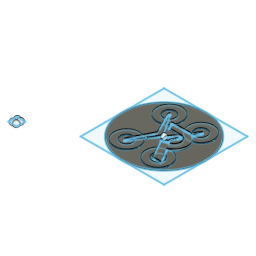
2023_02_01_DroneXR Logo Fusion360 v2 (Autodesk Fusion 360 design; units mm, degrees)
Autodesk Fusion 360 part; units mm, degrees
sketch "Esquisse1" plane through (0, 0, 0) normal (0, 0, 1) x (1, 0, 0)
  circle A0 centre (-3.2921, 4.4307) radius 1.2456
  circle A1 centre (-3.272, 4.4103) radius 2.5804
  circle A2 centre (3.328, 4.4103) radius 2.5804
  circle A3 centre (3.3079, 4.4307) radius 1.2456
  circle A4 centre (3.3079, -4.5693) radius 1.2456
  circle A5 centre (3.328, -4.5897) radius 2.5804
  circle A6 centre (-3.272, -4.5897) radius 2.5804
  circle A7 centre (-3.2921, -4.5693) radius 1.2456
  dimension "d1" = 5.1608
  dimension "d2" = 5.1608
  dimension "d3" = 5.1608
  dimension "d4" = 5.1608
  measures "d1" diameter of A1
  measures "d2" diameter of A2
  measures "d3" diameter of A6
  measures "d4" diameter of A5
sketch "Esquisse2" plane through (0, 0, 0) normal (0, 0, 1) x (1, 0, 0)
sketch "Esquisse3" plane through (0, 0, 0) normal (0, 0, 1) x (1, 0, 0)
  line L0 (-8.834, 8.7092) -> (9, 8.7092)
  line L1 (9, 8.7092) -> (9, -9)
  line L2 (9, -9) -> (-8.834, -9)
  line L3 (-8.834, -9) -> (-8.834, 8.7092)
  constraint horizontal L0
  constraint vertical L1
  constraint horizontal L2
  constraint vertical L3
extrude "Extrusion1" add sketch "Esquisse3" along normal blind 1 makes body 1
sketch "Esquisse4" plane through (0, 0, 1) normal (0, 0, 1) x (1, 0, 0)
  line L0 (163.6647, 105.2472) -> (164.171, 106.2352)
  line L1 (168.4405, 114.5503) -> (169.3629, 116.3496)
  line L2 (172.2245, 121.9555) -> (172.5459, 122.5884)
  line L3 (163.1727, 104.2862) -> (163.6647, 105.2472)
  line L4 (162.6946, 103.3518) -> (163.1727, 104.2862)
  line L5 (165.7765, 109.3648) -> (166.3413, 110.4645)
  line L6 (164.171, 106.2352) -> (164.6915, 107.2505)
  line L7 (169.3629, 116.3496) -> (169.8158, 117.2344)
  line L8 (169.8158, 117.2344) -> (170.2592, 118.1011)
  line L9 (170.2592, 118.1011) -> (170.6898, 118.944)
  line L10 (171.5009, 120.5336) -> (171.8752, 121.2685)
  line L11 (171.1047, 119.7568) -> (171.5009, 120.5336)
  line L12 (164.6915, 107.2505) -> (165.2267, 108.2936)
  line L13 (166.3413, 110.4645) -> (166.9213, 111.5932)
  line L14 (170.6898, 118.944) -> (171.1047, 119.7568)
  line L15 (165.2267, 108.2936) -> (165.7765, 109.3648)
  line L16 (167.5165, 112.7512) -> (168.4405, 114.5503)
  line L17 (171.8752, 121.2685) -> (172.2245, 121.9555)
  line L18 (166.9213, 111.5932) -> (167.5165, 112.7512)
  line L19 (169.7379, 137.8689) -> (169.0151, 139.2846)
  line L20 (158.4614, 160.0548) -> (158.1062, 160.7629)
  line L21 (156.2644, 164.4652) -> (156.0029, 164.9969)
  line L22 (158.8311, 159.3192) -> (158.4614, 160.0548)
  line L23 (175.0197, 127.5244) -> (169.7379, 137.8689)
  line L24 (156.0029, 164.9969) -> (155.7536, 165.5058)
  line L25 (153.887, 175.9712) -> (153.9857, 175.8402)
  line L26 (159.2157, 158.5552) -> (158.8311, 159.3192)
  line L27 (152.7535, 176.1782) -> (152.8565, 176.2955)
  line L28 (158.1062, 160.7629) -> (157.7652, 161.4439)
  line L29 (173.4904, 124.4603) -> (175.0197, 127.5244)
  line L30 (155.2906, 166.4578) -> (154.8728, 167.3261)
  line L31 (165.0973, 146.9651) -> (164.5114, 148.1152)
  line L32 (156.8251, 163.331) -> (156.5384, 163.9101)
  line L33 (156.5384, 163.9101) -> (156.2644, 164.4652)
  line L34 (168.3127, 140.6606) -> (167.6305, 141.9974)
  line L35 (162.8629, 151.3547) -> (162.3489, 152.3664)
  line L36 (172.5459, 122.5884) -> (172.8363, 123.1614)
  line L37 (157.7652, 161.4439) -> (157.4383, 162.0986)
  line L38 (157.4383, 162.0986) -> (157.125, 162.7274)
  line L39 (155.7536, 165.5058) -> (155.5163, 165.9926)
  line L40 (160.9087, 155.2051) -> (160.4617, 156.088)
  line L41 (161.372, 154.291) -> (160.9087, 155.2051)
  line L42 (152.4093, 174.3945) -> (152.4147, 174.7456)
  line L43 (172.8363, 123.1614) -> (173.0925, 123.6683)
  line L44 (159.6155, 157.7625) -> (159.2157, 158.5552)
  line L45 (173.0925, 123.6683) -> (173.3116, 124.1033)
  line L46 (161.852, 153.3449) -> (161.372, 154.291)
  line L47 (167.6305, 141.9974) -> (166.9681, 143.2957)
  line L48 (166.3253, 144.5559) -> (165.7018, 145.7789)
  line L49 (162.3489, 152.3664) -> (161.852, 153.3449)
  line L50 (163.9439, 149.2297) -> (163.3945, 150.3094)
  line L51 (160.4617, 156.088) -> (160.0307, 156.9403)
  line L52 (153.0203, 171.4671) -> (152.8804, 171.8403)
  line L53 (224.1626, 173.5518) -> (224.0834, 173.0993)
  line L54 (157.125, 162.7274) -> (156.8251, 163.331)
  line L55 (166.9681, 143.2957) -> (166.3253, 144.556)
  line L56 (155.5163, 165.9926) -> (155.2906, 166.4578)
  line L57 (154.8729, 167.3261) -> (154.4981, 168.1155)
  line L58 (169.0151, 139.2846) -> (168.3127, 140.6606)
  line L59 (160.0307, 156.9403) -> (159.6155, 157.7625)
  line L60 (165.7018, 145.7789) -> (165.0973, 146.9651)
  line L61 (164.5114, 148.1152) -> (163.9439, 149.2297)
  line L62 (173.3116, 124.1033) -> (173.4904, 124.4603)
  line L63 (163.3945, 150.3094) -> (162.8629, 151.3547)
  line L64 (152.4197, 174.0139) -> (152.4093, 174.3945)
  line L65 (153.8079, 176.0723) -> (153.887, 175.9712)
  line L66 (154.2397, 175.492) -> (154.3938, 175.2765)
  line L67 (223.966, 172.605) -> (223.8091, 172.0654)
  line L68 (153.6081, 170.0588) -> (153.3818, 170.5812)
  line L69 (152.671, 172.4716) -> (152.5966, 172.7394)
  line L70 (224.2047, 173.9663) -> (224.1626, 173.5518)
  line L71 (154.1035, 175.6802) -> (154.2397, 175.492)
  line L72 (152.4147, 174.7456) -> (152.4355, 175.0662)
  line L73 (223.6117, 171.4766) -> (223.3725, 170.835)
  line L74 (159.2102, 168.2167) -> (159.9788, 167.0685)
  line L75 (223.3725, 170.835) -> (223.0905, 170.1367)
  line L76 (152.4464, 173.6048) -> (152.4197, 174.0139)
  line L77 (223.0905, 170.1367) -> (222.7643, 169.378)
  line L78 (154.4981, 168.1155) -> (154.164, 168.8308)
  line L79 (152.5214, 175.6122) -> (152.5854, 175.8355)
  line L80 (152.5854, 175.8355) -> (152.663, 176.0245)
  line L81 (153.0982, 176.4172) -> (153.2358, 176.4197)
  line L82 (152.9716, 176.3755) -> (153.0982, 176.4172)
  line L83 (152.4967, 173.2035) -> (152.4464, 173.6048)
  line L84 (155.178, 174.1567) -> (155.4132, 173.8165)
  line L85 (154.3938, 175.2765) -> (154.5652, 175.0343)
  line L86 (154.9579, 174.4736) -> (155.178, 174.1567)
  line L87 (222.7643, 169.378) -> (222.3929, 168.5553)
  line L88 (155.9267, 173.0696) -> (156.4938, 172.2394)
  line L89 (152.7648, 172.1735) -> (152.671, 172.4716)
  line L90 (153.9857, 175.8402) -> (154.1035, 175.6802)
  line L91 (160.7744, 165.8763) -> (161.5923, 164.6467)
  line L92 (153.3841, 176.3819) -> (153.5425, 176.3029)
  line L93 (156.4938, 172.2394) -> (157.1102, 171.3324)
  line L94 (157.7714, 170.3553) -> (158.4729, 169.3145)
  line L95 (152.4355, 175.0662) -> (152.4712, 175.3554)
  line L96 (155.4132, 173.8165) -> (155.9267, 173.0696)
  line L97 (159.9788, 167.0685) -> (160.7744, 165.8763)
  line L98 (157.1102, 171.3324) -> (157.7714, 170.3553)
  line L99 (153.2358, 176.4197) -> (153.3841, 176.3819)
  line L100 (153.7488, 176.1428) -> (153.8079, 176.0723)
  line L101 (154.5652, 175.0343) -> (154.7535, 174.7664)
  line L102 (152.663, 176.0245) -> (152.7535, 176.1782)
  line L103 (153.3818, 170.5812) -> (153.1866, 171.049)
  line L104 (218.717, 161.3608) -> (218.4584, 161.0444)
  line L105 (154.7535, 174.7664) -> (154.9579, 174.4736)
  line L106 (152.4712, 175.3554) -> (152.5214, 175.6122)
  line L107 (153.7105, 176.1818) -> (153.7488, 176.1428)
  line L108 (224.1826, 174.6965) -> (224.211, 174.3467)
  line L109 (153.1866, 171.049) -> (153.0203, 171.4671)
  line L110 (217.6792, 160.635) -> (217.3833, 160.654)
  line L111 (153.5425, 176.3029) -> (153.7105, 176.1818)
  line L112 (158.4729, 169.3145) -> (159.2102, 168.2167)
  line L113 (161.5923, 164.6467) -> (162.4282, 163.3863)
  line L114 (152.5966, 172.7394) -> (152.4967, 173.2035)
  line L115 (153.8681, 169.477) -> (153.6081, 170.0588)
  line L116 (224.0262, 175.3196) -> (224.1206, 175.0196)
  line L117 (219.6742, 171.3631) -> (220.1184, 172.0026)
  line L118 (224.211, 174.3467) -> (224.2047, 173.9663)
  line L119 (224.0834, 173.0993) -> (223.966, 172.605)
  line L120 (152.8565, 176.2955) -> (152.9716, 176.3755)
  line L121 (215.1574, 161.5826) -> (213.5466, 162.3277)
  line L122 (220.5449, 172.6114) -> (220.951, 173.1861)
  line L123 (224.1206, 175.0196) -> (224.1826, 174.6965)
  line L124 (221.975, 167.6647) -> (221.5095, 166.7027)
  line L125 (223.8091, 172.0654) -> (223.6117, 171.4766)
  line L126 (223.8592, 175.6869) -> (224.0262, 175.3196)
  line L127 (220.7264, 165.1271) -> (220.4764, 164.6246)
  line L128 (223.0053, 175.951) -> (223.155, 176.1234)
  line L129 (152.8804, 171.8403) -> (152.7648, 172.1735)
  line L130 (154.164, 168.8308) -> (153.8681, 169.477)
  line L131 (220.2437, 164.1569) -> (220.0272, 163.723)
  line L132 (218.2062, 160.8228) -> (217.95, 160.6888)
  line L133 (221.3341, 173.723) -> (221.6917, 174.2185)
  line L134 (223.261, 176.2295) -> (223.3207, 176.2656)
  line L135 (219.6372, 162.9533) -> (219.4611, 162.6155)
  line L136 (218.2607, 169.2967) -> (218.7427, 170.0066)
  line L137 (217.95, 160.6888) -> (217.6792, 160.635)
  line L138 (222.585, 175.4213) -> (222.8144, 175.7157)
  line L139 (223.3975, 176.2463) -> (223.4833, 176.191)
  line L140 (216.2392, 161.0739) -> (215.7372, 161.3103)
  line L141 (219.1402, 162.0295) -> (218.9927, 161.7795)
  line L142 (219.2147, 170.6966) -> (219.6742, 171.3631)
  line L143 (221.6917, 174.2185) -> (222.0211, 174.6691)
  line L144 (223.6706, 175.9877) -> (223.8592, 175.6869)
  line L145 (221.5095, 166.7027) -> (220.9953, 165.6653)
  line L146 (218.7427, 170.0066) -> (219.2147, 170.6966)
  line L147 (222.8144, 175.7157) -> (223.0053, 175.951)
  line L148 (223.4833, 176.191) -> (223.5753, 176.1035)
  line L149 (220.951, 173.1861) -> (221.3341, 173.723)
  line L150 (220.4764, 164.6246) -> (220.2437, 164.1569)
  line L151 (218.9927, 161.7795) -> (218.852, 161.5569)
  line L152 (217.3833, 160.654) -> (217.0516, 160.7384)
  line L153 (220.0272, 163.723) -> (219.8255, 163.3221)
  line L154 (220.9953, 165.6653) -> (220.7264, 165.1271)
  line L155 (219.4611, 162.6155) -> (219.2959, 162.3079)
  line L156 (215.7372, 161.3103) -> (215.1574, 161.5826)
  line L157 (223.3207, 176.2656) -> (223.3975, 176.2463)
  line L158 (222.0211, 174.6691) -> (222.3197, 175.0712)
  line L159 (222.3929, 168.5553) -> (221.975, 167.6647)
  line L160 (217.0516, 160.7384) -> (216.6738, 160.8808)
  line L161 (222.3197, 175.0712) -> (222.5851, 175.4213)
  line L162 (218.4584, 161.0444) -> (218.2062, 160.8228)
  line L163 (213.5466, 162.3277) -> (218.2607, 169.2967)
  line L164 (216.6738, 160.8808) -> (216.2392, 161.0739)
  line L165 (220.1184, 172.0026) -> (220.5449, 172.6114)
  line L166 (223.155, 176.1234) -> (223.261, 176.2295)
  line L167 (223.5753, 176.1035) -> (223.6706, 175.9877)
  line L168 (219.8255, 163.3221) -> (219.6372, 162.9532)
  line L169 (218.852, 161.5569) -> (218.717, 161.3608)
  line L170 (219.2959, 162.3079) -> (219.1402, 162.0295)
  line L171 (226.9033, 88.3318) -> (227.2681, 87.7236)
  line L172 (222.1093, 156.076) -> (222.1115, 156.0742)
  line L173 (229.0186, 84.7682) -> (229.1794, 84.4974)
  line L174 (229.7465, 83.5555) -> (230.1781, 82.847)
  line L175 (231.1091, 81.3361) -> (232.0404, 79.8471)
  line L176 (216.8371, 104.8931) -> (216.9864, 104.6566)
  line L177 (219.9288, 99.8599) -> (220.3805, 99.1177)
  line L178 (227.9081, 86.6529) -> (228.1775, 86.2)
  line L179 (216.4685, 105.4941) -> (216.8371, 104.8931)
  line L180 (215.9806, 106.7639) -> (215.9168, 106.6982)
  line L181 (217.4117, 103.9725) -> (217.682, 103.5343)
  line L182 (215.8945, 106.6574) -> (215.9122, 106.5723)
  line L183 (226.5126, 88.9823) -> (226.9033, 88.3318)
  line L184 (228.1775, 86.2) -> (228.4095, 85.8085)
  line L185 (220.3805, 99.1177) -> (220.8467, 98.3511)
  line L186 (222.7974, 95.136) -> (223.784, 93.5059)
  line L187 (227.6039, 87.1624) -> (227.9081, 86.6529)
  line L188 (216.0528, 106.2499) -> (216.1679, 106.027)
  line L189 (221.8105, 96.7638) -> (222.7974, 95.136)
  line L190 (215.9168, 106.6982) -> (215.8945, 106.6574)
  line L191 (228.601, 85.4829) -> (228.7493, 85.2282)
  line L192 (219.4943, 100.573) -> (219.9288, 99.8599)
  line L193 (218.6887, 101.8926) -> (219.08, 101.2521)
  line L194 (229.3555, 84.2032) -> (229.7465, 83.5555)
  line L195 (226.0988, 89.6702) -> (226.5126, 88.9823)
  line L196 (229.1794, 84.4974) -> (229.3555, 84.2032)
  line L197 (202.7538, 99.6614) -> (201.9677, 101.0015)
  line L198 (227.2681, 87.7236) -> (227.6039, 87.1624)
  arc A0 (214.7629, 79.2757) -> (208.7557, 89.4625) centre (-17229.0104, -10200.5977) ccw
  line L199 (196.5103, 110.3428) -> (195.947, 111.3124)
  line L200 (194.8163, 119.1078) -> (195.4814, 119.1331)
  line L201 (230.1781, 82.847) -> (231.1091, 81.3361)
  line L202 (224.7475, 91.9115) -> (225.2134, 91.1396)
  line L203 (205.2271, 95.4521) -> (204.3845, 96.885)
  line L204 (218.5038, 76.1852) -> (216.7108, 75.9697)
  line L205 (217.1789, 104.3482) -> (217.4117, 103.9725)
  line L206 (191.688, 118.7768) -> (191.6308, 118.8958)
  line L207 (215.9663, 106.4341) -> (216.0528, 106.2499)
  line L208 (193.6407, 119.06) -> (194.2012, 119.0833)
  line L209 (206.9617, 92.5056) -> (206.0865, 93.9918)
  line L210 (201.9677, 101.0015) -> (201.2023, 102.3072)
  line L211 (199.4034, 119.2664) -> (200.276, 119.2932)
  line L212 (228.8746, 85.0127) -> (229.0186, 84.7682)
  line L213 (218.3234, 102.4896) -> (218.6887, 101.8926)
  line L214 (220.8467, 98.3511) -> (221.8105, 96.7638)
  line L215 (200.276, 119.2932) -> (208.8366, 119.5514)
  line L216 (215.9122, 106.5723) -> (215.9663, 106.4341)
  line L217 (192.891, 116.6136) -> (192.5931, 117.1381)
  line L218 (191.7878, 118.5859) -> (191.688, 118.7768)
  line L219 (225.2134, 91.1396) -> (225.6647, 90.3909)
  line L220 (216.1679, 106.027) -> (216.4685, 105.4941)
  line L221 (224.4113, 76.3855) -> (223.064, 76.3651)
  line L222 (193.2256, 116.0275) -> (192.891, 116.6136)
  line L223 (193.5958, 115.3815) -> (193.2256, 116.0275)
  line L224 (192.3329, 117.5993) -> (192.1112, 117.9955)
  line L225 (196.9443, 119.1856) -> (197.7332, 119.2124)
  line L226 (216.7108, 75.9697) -> (214.7629, 79.2757)
  line L227 (207.8518, 90.9952) -> (206.9617, 92.5056)
  line L228 (197.1024, 109.3251) -> (196.5103, 110.3428)
  line L229 (200.4588, 103.5769) -> (199.738, 104.8089)
  line L230 (232.0404, 79.8471) -> (234.2115, 76.4068)
  line L231 (192.5931, 117.1381) -> (192.3329, 117.5993)
  line L232 (217.9868, 103.0385) -> (218.3234, 102.4896)
  line L233 (228.7493, 85.2282) -> (228.8746, 85.0127)
  line L234 (234.2115, 76.4068) -> (227.2542, 76.4037)
  line L235 (217.682, 103.5343) -> (217.9868, 103.0385)
  line L236 (228.4095, 85.8085) -> (228.601, 85.4829)
  line L237 (223.784, 93.5059) -> (224.7475, 91.9115)
  line L238 (222.5957, 111.1484) -> (222.5957, 111.1484)
  line L239 (219.08, 101.2521) -> (219.4943, 100.573)
  line L240 (194.0006, 114.6773) -> (193.5958, 115.3815)
  line L241 (216.9864, 104.6566) -> (217.1789, 104.3482)
  line L242 (225.6647, 90.3909) -> (226.0988, 89.6702)
  line L243 (198.3687, 107.1527) -> (197.7222, 108.2612)
  line L244 (192.0329, 118.9807) -> (192.3308, 118.9981)
  line L245 (194.0711, 161.5559) -> (195.3383, 161.5737)
  line L246 (199.738, 104.8089) -> (199.041, 106.0014)
  line L247 (177.1219, 161.4007) -> (178.1749, 161.4193)
  line L248 (196.1923, 119.1591) -> (196.9443, 119.1856)
  line L249 (206.0865, 93.9918) -> (205.2271, 95.4521)
  line L250 (199.041, 106.0014) -> (198.3687, 107.1527)
  line L251 (219.749, 76.2691) -> (219.3497, 76.2492)
  line L252 (194.2012, 119.0833) -> (194.8163, 119.1078)
  line L253 (178.3207, 149.9378) -> (178.1604, 150.2288)
  line L254 (219.006, 76.2285) -> (218.7226, 76.2071)
  line L255 (193.1392, 119.0379) -> (193.6407, 119.06)
  line L256 (220.1996, 76.288) -> (219.749, 76.2691)
  line L257 (172.5687, 161.2483) -> (172.7534, 161.2614)
  line L258 (191.6308, 118.8958) -> (191.6172, 118.9413)
  line L259 (194.4392, 113.9166) -> (194.0006, 114.6773)
  line L260 (191.8117, 118.9654) -> (192.0329, 118.9807)
  line L261 (195.947, 111.3124) -> (195.4134, 112.2324)
  line L262 (191.6172, 118.9413) -> (191.6716, 118.9522)
  line L263 (204.3845, 96.885) -> (203.5598, 98.2887)
  line L264 (223.064, 76.3651) -> (221.8139, 76.3382)
  line L265 (191.9292, 118.3249) -> (191.7878, 118.5859)
  line L266 (192.3308, 118.9981) -> (192.7011, 119.0172)
  line L267 (225.82, 76.3987) -> (224.4113, 76.3855)
  line L268 (192.7011, 119.0172) -> (193.1392, 119.0379)
  line L269 (218.7226, 76.2071) -> (218.5038, 76.1852)
  line L270 (221.8139, 76.3382) -> (221.2365, 76.3227)
  line L271 (191.6716, 118.9522) -> (191.8117, 118.9654)
  line L272 (197.7222, 108.2612) -> (197.1024, 109.3251)
  line L273 (195.4814, 119.1331) -> (196.1923, 119.1591)
  line L274 (192.1112, 117.9955) -> (191.9292, 118.3249)
  line L275 (220.6969, 76.3059) -> (220.1996, 76.288)
  line L276 (219.3497, 76.2492) -> (219.006, 76.2285)
  line L277 (194.9104, 113.101) -> (194.4392, 113.9166)
  line L278 (197.7332, 119.2124) -> (198.5543, 119.2394)
  line L279 (227.2542, 76.4037) -> (225.82, 76.3987)
  line L280 (195.4134, 112.2324) -> (194.9104, 113.101)
  line L281 (198.5543, 119.2394) -> (199.4034, 119.2664)
  line L282 (221.2365, 76.3227) -> (220.6969, 76.3059)
  line L283 (208.7557, 89.4625) -> (207.8518, 90.9952)
  line L284 (201.2023, 102.3072) -> (200.4588, 103.5769)
  line L285 (203.5598, 98.2887) -> (202.7538, 99.6614)
  line L286 (193.797, 147.6841) -> (179.5416, 147.6841)
  line L287 (185.805, 161.4888) -> (188.6273, 161.5026)
  line L288 (180.4964, 161.4512) -> (181.7509, 161.464)
  line L289 (173.7915, 161.3121) -> (174.1215, 161.3242)
  line L290 (192.7575, 161.5397) -> (194.0711, 161.5559)
  line L291 (173.1381, 159.2178) -> (172.9437, 159.5778)
  line L292 (172.9437, 159.5778) -> (172.7668, 159.9083)
  line L293 (172.969, 161.2743) -> (173.2144, 161.2871)
  line L294 (172.7668, 159.9083) -> (172.6089, 160.2069)
  line L295 (173.574, 158.4203) -> (173.3486, 158.8311)
  line L296 (177.33, 151.7233) -> (177.0846, 152.1627)
  line L297 (191.4064, 161.5254) -> (192.7575, 161.5397)
  line L298 (172.1948, 161.0294) -> (172.1526, 161.129)
  line L299 (172.4157, 161.235) -> (172.5687, 161.2483)
  line L300 (172.2082, 161.2081) -> (172.2952, 161.2216)
  line L301 (174.8725, 156.095) -> (174.3243, 157.0689)
  line L302 (173.2144, 161.2871) -> (173.4889, 161.2997)
  line L303 (176.1501, 161.3806) -> (177.1219, 161.4007)
  line L304 (176.5616, 153.0966) -> (176.0085, 154.0813)
  line L305 (183.0585, 161.4747) -> (184.4122, 161.483)
  line L306 (173.8126, 157.9879) -> (173.574, 158.4203)
  line L307 (172.6089, 160.2069) -> (172.4713, 160.4709)
  line L308 (175.2664, 161.3589) -> (176.1501, 161.3806)
  line L309 (172.1526, 161.129) -> (172.1379, 161.1809)
  line L310 (179.5416, 147.6841) -> (178.5713, 149.4789)
  line L311 (178.4583, 149.6867) -> (178.3207, 149.9378)
  line L312 (177.0846, 152.1627) -> (176.5616, 153.0966)
  line L313 (174.1215, 161.3242) -> (174.4779, 161.3361)
  line L314 (177.9793, 150.5562) -> (177.7792, 150.9167)
  line L315 (173.3487, 158.8311) -> (173.1381, 159.2178)
  line L316 (173.4889, 161.2997) -> (173.7915, 161.3121)
  line L317 (178.1749, 161.4193) -> (179.3021, 161.4362)
  line L318 (177.7792, 150.9167) -> (177.5622, 151.3069)
  line L319 (174.3243, 157.0689) -> (173.8126, 157.9879)
  line L320 (195.3383, 161.5737) -> (196.5501, 161.5929)
  line L321 (172.4713, 160.4709) -> (172.3555, 160.6978)
  line L322 (184.4122, 161.483) -> (185.805, 161.4888)
  line L323 (178.5713, 149.4789) -> (178.4583, 149.6867)
  line L324 (178.1604, 150.2288) -> (177.9793, 150.5562)
  line L325 (175.4404, 155.0898) -> (174.8725, 156.095)
  line L326 (172.3555, 160.6978) -> (172.2629, 160.8848)
  line L327 (181.7509, 161.464) -> (183.0585, 161.4747)
  line L328 (172.2629, 160.8848) -> (172.1948, 161.0294)
  line L329 (172.1379, 161.1809) -> (172.1554, 161.1946)
  line L330 (208.0524, 147.6841) -> (193.797, 147.6841)
  line L331 (172.1554, 161.1946) -> (172.2082, 161.2081)
  line L332 (176.0085, 154.0813) -> (175.4404, 155.0898)
  line L333 (172.7534, 161.2614) -> (172.969, 161.2743)
  line L334 (172.2952, 161.2216) -> (172.4157, 161.235)
  line L335 (177.5622, 151.3069) -> (177.33, 151.7233)
  line L336 (179.3021, 161.4362) -> (180.4964, 161.4511)
  line L337 (203.5703, 122.4171) -> (203.3147, 122.3953)
  line L338 (200.0392, 122.2837) -> (198.9757, 122.2783)
  line L339 (191.9008, 126.4962) -> (191.8147, 127.2457)
  line L340 (201.0796, 161.694) -> (201.4673, 161.7063)
  line L341 (208.3592, 162.0749) -> (208.7907, 162.0839)
  line L342 (202.3163, 122.339) -> (201.9151, 122.3237)
  line L343 (206.6371, 161.9991) -> (207.2866, 162.0325)
  line L344 (201.4673, 161.7063) -> (201.8277, 161.7187)
  line L345 (210.074, 162.01) -> (210.1859, 161.9717)
  line L346 (207.8592, 162.0577) -> (208.3592, 162.0749)
  line L347 (204.1359, 122.516) -> (204.0683, 122.4898)
  line L348 (208.2588, 140.4356) -> (208.0552, 140.0209)
  line L349 (208.4402, 140.8074) -> (208.2588, 140.4356)
  line L350 (207.3325, 138.5613) -> (207.0612, 138.0169)
  line L351 (198.9757, 122.2783) -> (193.668, 122.2783)
  line L352 (209.9196, 162.0405) -> (210.074, 162.01)
  line L353 (201.8277, 161.7187) -> (202.1599, 161.7313)
  line L354 (192.7247, 124.1308) -> (192.3558, 124.9384)
  line L355 (203.3147, 122.3953) -> (203.0188, 122.3749)
  line L356 (202.9755, 161.7696) -> (203.1833, 161.7825)
  line L357 (202.7349, 161.7568) -> (202.9755, 161.7696)
  line L358 (203.1833, 161.7825) -> (204.1837, 161.8492)
  line L359 (197.6977, 161.6135) -> (198.7721, 161.6353)
  line L360 (174.4779, 161.3361) -> (175.2664, 161.3589)
  line L361 (205.0899, 161.9075) -> (205.9063, 161.9574)
  line L362 (203.0188, 122.3749) -> (202.685, 122.3561)
  line L363 (207.2866, 162.0325) -> (207.8592, 162.0577)
  line L364 (209.8624, 143.7944) -> (208.7282, 141.4055)
  line L365 (201.6983, 127.4328) -> (202.8572, 125.1202)
  line L366 (200.6658, 161.6818) -> (201.0796, 161.694)
  line L367 (209.1583, 162.0849) -> (209.4661, 162.078)
  line L368 (208.7907, 162.0839) -> (209.1583, 162.0849)
  line L369 (204.6462, 133.2246) -> (201.6983, 127.4328)
  line L370 (208.5973, 141.1321) -> (208.4402, 140.8074)
  line L371 (204.1837, 161.8492) -> (205.0899, 161.9075)
  line L372 (207.8315, 139.5675) -> (207.5899, 139.0796)
  line L373 (201.4841, 122.3104) -> (201.0261, 122.2992)
  line L374 (201.0261, 122.2992) -> (200.0392, 122.2837)
  line L375 (193.668, 122.2783) -> (192.7247, 124.1308)
  line L376 (205.9063, 161.9574) -> (206.6371, 161.9991)
  line L377 (204.0683, 122.4898) -> (203.9498, 122.4645)
  arc A1 (202.8572, 125.1202) -> (204.1498, 122.543) centre (974.9031, 510.7212) ccw
  line L378 (202.1599, 161.7313) -> (202.4627, 161.744)
  line L379 (202.6851, 122.3561) -> (202.3163, 122.339)
  line L380 (188.6273, 161.5026) -> (191.4064, 161.5254)
  line L381 (209.7184, 162.0632) -> (209.9197, 162.0405)
  line L382 (202.4627, 161.744) -> (202.7349, 161.7568)
  line L383 (196.5501, 161.5929) -> (197.6977, 161.6135)
  line L384 (207.5899, 139.0796) -> (207.3325, 138.5613)
  line L385 (209.4661, 162.078) -> (209.7184, 162.0632)
  line L386 (205.8802, 135.662) -> (204.6462, 133.2246)
  line L387 (208.7282, 141.4055) -> (208.5973, 141.1321)
  line L388 (204.1498, 122.543) -> (204.1359, 122.516)
  line L389 (203.9498, 122.4645) -> (203.7829, 122.4402)
  line L390 (198.7721, 161.6353) -> (199.7644, 161.6581)
  line L391 (203.7829, 122.4402) -> (203.5703, 122.4171)
  line L392 (208.0552, 140.0209) -> (207.8316, 139.5675)
  line L393 (207.0612, 138.0169) -> (205.8802, 135.662)
  line L394 (201.9151, 122.3237) -> (201.4841, 122.3104)
  line L395 (192.3558, 124.9384) -> (192.0812, 125.727)
  line L396 (195.0358, 134.222) -> (195.4588, 134.8733)
  line L397 (205.8598, 145.5476) -> (206.1334, 145.5309)
  line L398 (193.9038, 132.4625) -> (194.2556, 133.0124)
  line L399 (193.0347, 131.0846) -> (193.2906, 131.4943)
  line L400 (192.4137, 130.0412) -> (192.5031, 130.2041)
  line L401 (195.8999, 135.5497) -> (196.8257, 136.961)
  line L402 (192.8163, 130.7301) -> (193.0347, 131.0846)
  line L403 (197.7911, 138.4216) -> (202.5328, 145.567)
  line L404 (192.0812, 125.727) -> (191.9008, 126.4962)
  line L405 (204.8933, 145.567) -> (205.2422, 145.565)
  line L406 (207.0511, 145.3969) -> (207.4389, 145.2811)
  line L407 (194.6339, 133.6003) -> (195.0358, 134.222)
  line L408 (206.6225, 145.4785) -> (207.0511, 145.3969)
  line L409 (183.6889, 131.0836) -> (183.8612, 130.806)
  line L410 (192.6382, 130.4351) -> (192.8163, 130.7301)
  line L411 (192.5031, 130.2041) -> (192.6382, 130.4351)
  line L412 (199.7644, 161.6581) -> (200.6658, 161.6819)
  line L413 (202.5328, 145.567) -> (204.8933, 145.567)
  line L414 (206.1334, 145.5309) -> (206.6225, 145.4785)
  line L415 (170.0216, 151.9137) -> (170.6134, 151.0188)
  line L416 (208.558, 144.6807) -> (209.8624, 143.7944)
  line L417 (184.2074, 130.2251) -> (184.2709, 130.1079)
  line L418 (192.1224, 129.3733) -> (192.4137, 130.0412)
  line L419 (184.2709, 130.1079) -> (184.4283, 129.7709)
  line L420 (167.4946, 155.7333) -> (168.1507, 154.7418)
  line L421 (205.5636, 145.5588) -> (205.8598, 145.5476)
  line L422 (171.7504, 149.2991) -> (172.2959, 148.4737)
  line L423 (191.823, 127.9753) -> (191.9255, 128.6846)
  line L424 (193.2906, 131.4943) -> (193.5812, 131.9551)
  line L425 (205.2422, 145.565) -> (205.5636, 145.5587)
  line L426 (183.8612, 130.806) -> (184.0041, 130.5718)
  line L427 (178.0872, 139.6955) -> (178.7787, 138.6438)
  line L428 (194.2556, 133.0124) -> (194.6339, 133.6003)
  line L429 (193.5812, 131.9551) -> (193.9038, 132.4625)
  line L430 (207.4389, 145.2811) -> (207.806, 145.1264)
  line L431 (207.8061, 145.1264) -> (208.1725, 144.9278)
  line L432 (208.1724, 144.9278) -> (208.5581, 144.6807)
  line L433 (195.4588, 134.8733) -> (195.8999, 135.5497)
  line L434 (191.9255, 128.6846) -> (192.1224, 129.3733)
  line L435 (184.119, 130.3789) -> (184.2074, 130.2251)
  line L436 (191.8147, 127.2457) -> (191.823, 127.9753)
  line L437 (196.8257, 136.961) -> (197.7911, 138.4216)
  line L438 (182.8144, 122.2968) -> (182.5222, 121.842)
  line L439 (182.6753, 132.6755) -> (182.9803, 132.2008)
  line L440 (156.4772, 82.9931) -> (156.0798, 82.4174)
  line L441 (183.6666, 123.652) -> (183.5034, 123.3863)
  line L442 (184.8223, 127.0956) -> (184.711, 126.2769)
  line L443 (183.7946, 123.8662) -> (183.6666, 123.652)
  line L444 (158.3035, 85.6556) -> (157.8137, 84.9395)
  line L445 (153.8154, 79.2221) -> (153.7313, 79.1199)
  line L446 (153.5283, 78.9933) -> (153.3816, 78.9418)
  line L447 (184.0041, 130.5718) -> (184.119, 130.3789)
  line L448 (174.3295, 145.3952) -> (174.8017, 144.6799)
  line L449 (183.25, 131.7788) -> (183.4857, 131.4072)
  line L450 (176.5513, 142.0275) -> (177.3452, 140.8226)
  line L451 (166.822, 156.7497) -> (167.4946, 155.7333)
  line L452 (183.4857, 131.4072) -> (183.6889, 131.0836)
  line L453 (181.0705, 135.1469) -> (181.5324, 134.4386)
  line L454 (172.8264, 147.6709) -> (173.3421, 146.8904)
  line L455 (181.9528, 133.7922) -> (182.3332, 133.2052)
  line L456 (180.5657, 135.9193) -> (181.0705, 135.1469)
  line L457 (171.1896, 150.1474) -> (171.7504, 149.2991)
  line L458 (166.1326, 157.7912) -> (166.822, 156.7497)
  line L459 (153.7313, 79.1199) -> (153.6849, 79.0747)
  line L460 (177.3452, 140.8226) -> (178.0872, 139.6955)
  line L461 (184.8349, 127.9007) -> (184.841, 127.5006)
  line L462 (153.3816, 78.9418) -> (153.2449, 78.9202)
  line L463 (178.1814, 115.2262) -> (177.6314, 114.3964)
  line L464 (174.8017, 144.6799) -> (175.704, 143.3125)
  line L465 (156.0798, 82.4174) -> (155.7084, 81.8811)
  line L466 (175.704, 143.3125) -> (176.5513, 142.0275)
  line L467 (180.0165, 136.758) -> (180.5657, 135.9193)
  line L468 (184.1962, 124.6495) -> (183.7946, 123.8662)
  line L469 (170.6134, 151.0188) -> (171.1896, 150.1474)
  line L470 (172.2959, 148.4737) -> (172.8264, 147.6709)
  line L471 (182.9803, 132.2008) -> (183.25, 131.7788)
  line L472 (163.2041, 162.2147) -> (163.9622, 161.0697)
  line L473 (168.1507, 154.7418) -> (168.7904, 153.7749)
  line L474 (164.7029, 159.9509) -> (165.4263, 158.8582)
  line L475 (184.5602, 129.4195) -> (184.6667, 129.0552)
  line L476 (173.843, 146.132) -> (174.3295, 145.3952)
  line L477 (178.7787, 138.6438) -> (179.4213, 137.6655)
  line L478 (173.3421, 146.8904) -> (173.843, 146.132)
  line L479 (165.4263, 158.8582) -> (166.1326, 157.7912)
  line L480 (182.3332, 133.2052) -> (182.6753, 132.6756)
  line L481 (169.414, 152.8323) -> (170.0216, 151.9137)
  line L482 (184.841, 127.5006) -> (184.8223, 127.0956)
  line L483 (181.5324, 134.4386) -> (181.9528, 133.7922)
  line L484 (180.1942, 118.2748) -> (179.7215, 117.5568)
  line L485 (182.5222, 121.842) -> (182.2006, 121.3444)
  line L486 (159.3421, 87.1781) -> (158.8133, 86.4023)
  line L487 (163.9622, 161.0697) -> (164.7029, 159.9509)
  line L488 (179.4213, 137.6655) -> (180.0165, 136.7581)
  line L489 (162.4282, 163.3863) -> (163.2041, 162.2147)
  line L490 (168.7904, 153.7749) -> (169.414, 152.8323)
  line L491 (184.7479, 128.6796) -> (184.8039, 128.2942)
  line L492 (157.072, 92.255) -> (157.6655, 93.4421)
  line L493 (161.6234, 90.5355) -> (160.4519, 88.8094)
  line L494 (168.0767, 100.0977) -> (166.738, 98.1078)
  line L495 (154.7312, 87.4724) -> (155.1209, 88.2857)
  line L496 (173.3891, 108.0246) -> (170.7602, 104.0958)
  line L497 (179.2276, 116.8082) -> (178.7139, 116.0308)
  line L498 (153.6849, 79.0747) -> (153.5283, 78.9933)
  line L499 (184.502, 125.4573) -> (184.1962, 124.6495)
  line L500 (153.9363, 79.3796) -> (153.8154, 79.2221)
  line L501 (158.8133, 86.4023) -> (158.3035, 85.6556)
  line L502 (183.3062, 123.0706) -> (183.0761, 122.7069)
  line L503 (152.4981, 82.1439) -> (152.5734, 82.4119)
  line L504 (164.1138, 94.2161) -> (162.8472, 92.3424)
  line L505 (152.8944, 79.0345) -> (152.7974, 79.1322)
  line L506 (156.8994, 83.6065) -> (156.4772, 82.9931)
  line L507 (170.7602, 104.0958) -> (168.0767, 100.0977)
  line L508 (155.0484, 80.934) -> (154.7621, 80.5267)
  line L509 (174.6595, 109.928) -> (173.3891, 108.0246)
  line L510 (154.0587, 86.0386) -> (154.3776, 86.7244)
  line L511 (160.5073, 99.0642) -> (160.9183, 99.8717)
  line L512 (152.6336, 79.4167) -> (152.5668, 79.6036)
  line L513 (180.6447, 118.9604) -> (180.1942, 118.2748)
  line L514 (177.6314, 114.3964) -> (177.0651, 113.5429)
  line L515 (179.7215, 117.5568) -> (179.2276, 116.8082)
  line L516 (178.7139, 116.0308) -> (178.1814, 115.2262)
  line L517 (184.8039, 128.2942) -> (184.8349, 127.9007)
  line L518 (155.3642, 81.3861) -> (155.0484, 80.934)
  line L519 (184.4283, 129.7709) -> (184.5602, 129.4195)
  line L520 (175.8879, 111.7721) -> (174.6595, 109.928)
  line L521 (181.8509, 120.8057) -> (181.4742, 120.2276)
  line L522 (157.3453, 84.2559) -> (156.8994, 83.6065)
  line L523 (183.0761, 122.7069) -> (182.8144, 122.2968)
  line L524 (184.6667, 129.0552) -> (184.7479, 128.6796)
  line L525 (177.0651, 113.5429) -> (176.4835, 112.6676)
  line L526 (181.0718, 119.612) -> (180.6447, 118.9604)
  line L527 (154.283, 79.8532) -> (154.0925, 79.5905)
  line L528 (182.2006, 121.3444) -> (181.8509, 120.8057)
  line L529 (157.8137, 84.9395) -> (157.3453, 84.2559)
  line L530 (155.7084, 81.8811) -> (155.3642, 81.3861)
  line L531 (184.711, 126.2769) -> (184.502, 125.4573)
  line L532 (176.4835, 112.6676) -> (175.8879, 111.7721)
  line L533 (154.7621, 80.5267) -> (154.5066, 80.1658)
  line L534 (160.4519, 88.8094) -> (159.8887, 87.981)
  line L535 (154.0925, 79.5905) -> (153.9363, 79.3796)
  line L536 (162.8472, 92.3424) -> (161.6234, 90.5355)
  line L537 (159.8887, 87.981) -> (159.3421, 87.1781)
  line L538 (183.5034, 123.3863) -> (183.3062, 123.0706)
  line L539 (181.4742, 120.2276) -> (181.0718, 119.612)
  line L540 (153.773, 85.4117) -> (154.0587, 86.0386)
  line L541 (154.5066, 80.1658) -> (154.283, 79.8532)
  line L542 (165.4139, 96.1426) -> (164.1138, 94.2161)
  line L543 (156.015, 90.1208) -> (156.5224, 91.149)
  line L544 (166.738, 98.1078) -> (165.4139, 96.1426)
  line L545 (152.7974, 79.1322) -> (152.7105, 79.2596)
  line L546 (161.7796, 101.561) -> (162.2303, 102.4435)
  line L547 (152.3998, 80.6474) -> (152.3833, 80.9823)
  line L548 (160.1091, 98.2809) -> (160.5073, 99.0642)
  line L549 (159.7236, 97.5214) -> (160.1091, 98.2809)
  line L550 (152.6696, 82.7138) -> (152.7883, 83.0527)
  line L551 (152.5734, 82.4119) -> (152.6696, 82.7138)
  line L552 (153.5189, 84.8408) -> (153.773, 85.4117)
  line L553 (162.2303, 102.4435) -> (162.6946, 103.3518)
  line L554 (159.3505, 96.7852) -> (159.7236, 97.5214)
  line L555 (153.2449, 78.9202) -> (153.1181, 78.9285)
  line L556 (152.3833, 81.5111) -> (152.4046, 81.6966)
  line L557 (160.9183, 99.8717) -> (161.3424, 100.7039)
  line L558 (152.3833, 80.9823) -> (152.3768, 81.3468)
  line L559 (152.5099, 79.8201) -> (152.4631, 80.0662)
  line L560 (152.5668, 79.6036) -> (152.5099, 79.8201)
  line L561 (153.0994, 83.8539) -> (153.2948, 84.3226)
  line L562 (152.4631, 80.0662) -> (152.4264, 80.342)
  line L563 (152.4264, 80.342) -> (152.3998, 80.6474)
  line L564 (153.0012, 78.9666) -> (152.8944, 79.0345)
  line L565 (152.9311, 83.4317) -> (153.0994, 83.8539)
  line L566 (152.4046, 81.6966) -> (152.4424, 81.9065)
  line L567 (152.7883, 83.0527) -> (152.9311, 83.4317)
  line L568 (155.5483, 89.1675) -> (156.015, 90.1208)
  line L569 (158.3042, 94.7135) -> (158.641, 95.3817)
  line L570 (152.7105, 79.2596) -> (152.6336, 79.4167)
  line L571 (153.1181, 78.9285) -> (153.0012, 78.9666)
  line L572 (152.4424, 81.9065) -> (152.4981, 82.1439)
  line L573 (158.9897, 96.0722) -> (159.3505, 96.7852)
  line L574 (158.641, 95.3817) -> (158.9897, 96.0722)
  line L575 (154.3776, 86.7244) -> (154.7312, 87.4724)
  line L576 (152.3769, 81.3468) -> (152.3833, 81.5111)
  line L577 (161.3424, 100.7039) -> (161.7796, 101.561)
  line L578 (156.5224, 91.149) -> (157.072, 92.255)
  line L579 (153.2948, 84.3226) -> (153.5189, 84.8408)
  line L580 (155.1209, 88.2857) -> (155.5483, 89.1675)
  line L581 (157.6655, 93.4421) -> (158.3042, 94.7135)
  circle A2 centre (153.4724, 174.837) radius 12.9545
  circle A3 centre (153.4868, 175.0043) radius 26.7115
  circle A4 centre (221.4868, 175.0043) radius 26.7115
  circle A5 centre (221.4724, 174.837) radius 12.9545
  circle A6 centre (221.4724, 82.837) radius 12.9545
  circle A7 centre (221.4868, 83.0043) radius 26.7115
  circle A8 centre (153.4868, 83.0043) radius 26.7115
  circle A9 centre (153.4724, 82.837) radius 12.9545
  line L582 (97.5, 219.5) -> (277, 219.5)
  line L583 (277, 219.5) -> (277, 40)
  line L584 (277, 40) -> (97.5, 40)
  line L585 (97.5, 40) -> (97.5, 219.5)
  circle A10 centre (187.25, 129.75) radius 89.75
  spline S0 degree 5 poles (208.0524, 147.6841) (208.6483, 147.5213) (209.8038, 147.1664) (211.4285, 146.5466) (213.376, 145.5439) (215.4355, 143.9931) (217.1057, 142.1485) (218.3713, 140.0278) (219.22, 137.6723) (219.6482, 135.1572) (219.6584, 132.5794) (219.2569, 130.0429) (218.4533, 127.6455) (217.2599, 125.4652) (215.6938, 123.5458) (213.7725, 121.907) (211.9631, 120.8239) (210.4573, 120.1386) (209.3878, 119.7378) (208.8366, 119.5514) knots 0 0 0 0 0 0 0.066667 0.133333 0.2 0.266667 0.333333 0.4 0.466667 0.533333 0.6 0.666667 0.733333 0.8 0.866667 0.933333 1 1 1 1 1 1
  spline S1 degree 5 poles (210.1859, 161.9717) (210.6891, 161.8824) (211.6641, 161.675) (213.0324, 161.2775) (214.6974, 160.5988) (216.622, 159.5847) (218.1145, 158.6912) (219.2383, 157.9895) (219.9933, 157.5084) (220.3723, 157.2645) knots 0 0 0 0 0 0 0.2 0.4 0.6 0.8 1 1 1 1 1 1
  line L586 (219.3926, 157.8949) -> (221.3521, 156.6341)
  spline S2 degree 5 poles (222.1093, 156.076) (222.4153, 155.8533) (223.0674, 155.3656) (224.0487, 154.5868) (225.3274, 153.4725) (226.849, 151.9593) (228.3027, 150.2883) (229.6303, 148.5039) (230.8123, 146.6158) (231.8287, 144.6385) (232.6615, 142.5888) (233.2966, 140.4839) (233.7262, 138.3398) (233.9513, 136.1688) (233.9823, 133.9789) (233.8345, 131.7773) (233.5254, 129.5728) (233.0715, 127.3783) (232.4847, 125.2136) (231.7696, 123.107) (230.9275, 121.09) (229.9588, 119.1923) (228.8663, 117.4367) (227.6578, 115.8345) (226.3492, 114.3799) (225.0669, 113.1568) (224.0249, 112.2691) (223.2575, 111.6567) (222.7792, 111.288) (222.5957, 111.1484) knots 0.175139 0.175139 0.175139 0.175139 0.175139 0.175139 0.2 0.228571 0.257143 0.285714 0.314286 0.342857 0.371429 0.4 0.428571 0.457143 0.485714 0.514286 0.542857 0.571429 0.6 0.628571 0.657143 0.685714 0.714286 0.742857 0.771429 0.8 0.828571 0.857143 0.874848 0.874848 0.874848 0.874848 0.874848 0.874848
  line L587 (218.3046, 158.8438) -> (225.9139, 153.3082)
  line L588 (226.2412, 113.9223) -> (218.9502, 108.3744)
  spline S3 degree 5 poles (220.5972, 109.701) (220.5842, 109.692) (220.2701, 109.4748) (219.6537, 109.0551) (218.7325, 108.4466) (217.8085, 107.8606) (216.8954, 107.3041) (216.2857, 106.9424) (215.9806, 106.7639) knots 0.913051 0.913051 0.913051 0.913051 0.913051 0.913051 0.914286 0.942857 0.971429 1 1 1 1 1 1
  line L589 (221.0684, 110.0272) -> (220.1261, 109.3749)
  spline S4 degree 5 poles (222.1115, 156.0742) (222.042, 156.1218) (221.9028, 156.217) (221.6941, 156.3599) (221.4159, 156.5503) (221.068, 156.7884) (220.7897, 156.9788) (220.581, 157.1217) (220.4419, 157.2169) (220.3723, 157.2645) knots 0 0 0 0 0 0 0.2 0.4 0.6 0.8 1 1 1 1 1 1
  line L590 (208.5025, 144.5975) -> (209.7353, 143.7598)
  line L591 (209.7353, 143.7598) -> (208.6379, 141.4485)
  line L592 (208.6379, 141.4485) -> (208.5072, 141.1754)
  line L593 (208.5072, 141.1754) -> (208.3502, 140.8511)
  line L594 (208.3502, 140.8511) -> (208.1689, 140.4795)
  line L595 (208.1689, 140.4795) -> (207.9655, 140.065)
  line L596 (207.9655, 140.065) -> (207.7419, 139.6118)
  line L597 (207.7419, 139.6118) -> (207.5004, 139.124)
  line L598 (207.5004, 139.124) -> (207.2429, 138.6059)
  line L599 (207.2429, 138.6059) -> (206.9718, 138.0616)
  line L600 (206.9718, 138.0616) -> (205.7909, 135.7071)
  line L601 (205.7909, 135.7071) -> (204.557, 133.2699)
  line L602 (204.557, 133.2699) -> (201.5863, 127.4331)
  line L603 (201.5863, 127.4331) -> (202.7678, 125.0754)
  arc A11 (202.7678, 125.0754) -> (204.0184, 122.5814) centre (974.9031, 510.7212) ccw
  line L604 (204.0184, 122.5814) -> (203.9321, 122.563)
  line L605 (203.9321, 122.563) -> (203.7703, 122.5394)
  line L606 (203.7703, 122.5394) -> (203.5606, 122.5166)
  line L607 (203.5606, 122.5166) -> (203.307, 122.495)
  line L608 (203.307, 122.495) -> (203.0125, 122.4747)
  line L609 (203.0125, 122.4747) -> (202.6799, 122.4559)
  line L610 (202.6799, 122.4559) -> (202.3121, 122.4389)
  line L611 (202.3121, 122.4389) -> (201.9117, 122.4236)
  line L612 (201.9117, 122.4236) -> (201.4814, 122.4104)
  line L613 (201.4814, 122.4104) -> (201.0241, 122.3992)
  line L614 (201.0241, 122.3992) -> (200.0382, 122.3837)
  line L615 (200.0382, 122.3837) -> (198.9755, 122.3783)
  line L616 (198.9755, 122.3783) -> (193.7293, 122.3783)
  line L617 (193.7293, 122.3783) -> (192.8148, 124.1743)
  line L618 (192.8148, 124.1743) -> (192.4487, 124.9757)
  line L619 (192.4487, 124.9757) -> (192.1773, 125.7549)
  line L620 (192.1773, 125.7549) -> (191.9995, 126.5133)
  line L621 (191.9995, 126.5133) -> (191.9148, 127.2509)
  line L622 (191.9148, 127.2509) -> (191.9229, 127.9675)
  line L623 (191.9229, 127.9675) -> (192.0235, 128.6636)
  line L624 (192.0235, 128.6636) -> (192.2167, 129.3395)
  line L625 (192.2167, 129.3395) -> (192.5035, 129.9971)
  line L626 (192.5035, 129.9971) -> (192.5901, 130.1548)
  line L627 (192.5901, 130.1548) -> (192.7241, 130.384)
  line L628 (192.7241, 130.384) -> (192.9017, 130.678)
  line L629 (192.9017, 130.678) -> (193.1197, 131.0318)
  line L630 (193.1197, 131.0318) -> (193.3753, 131.4412)
  line L631 (193.3753, 131.4412) -> (193.6657, 131.9016)
  line L632 (193.6657, 131.9016) -> (193.9881, 132.4088)
  line L633 (193.9881, 132.4088) -> (194.3398, 132.9584)
  line L634 (194.3398, 132.9584) -> (194.7179, 133.5461)
  line L635 (194.7179, 133.5461) -> (195.1198, 134.1677)
  line L636 (195.1198, 134.1677) -> (195.5426, 134.8187)
  line L637 (195.5426, 134.8187) -> (195.9836, 135.495)
  line L638 (195.9836, 135.495) -> (196.9092, 136.906)
  line L639 (196.9092, 136.906) -> (197.8745, 138.3664)
  line L640 (197.8745, 138.3664) -> (202.5864, 145.467)
  line L641 (202.5864, 145.467) -> (204.893, 145.467)
  line L642 (204.893, 145.467) -> (205.241, 145.465)
  line L643 (205.241, 145.465) -> (205.5607, 145.4588)
  line L644 (205.5607, 145.4588) -> (205.8549, 145.4477)
  line L645 (205.8549, 145.4477) -> (206.125, 145.4312)
  line L646 (206.125, 145.4312) -> (206.6078, 145.3795)
  line L647 (206.6078, 145.3795) -> (207.0273, 145.2996)
  line L648 (207.0273, 145.2996) -> (207.4051, 145.1868)
  line L649 (207.4051, 145.1868) -> (207.7627, 145.0361)
  line L650 (207.7627, 145.0361) -> (208.1216, 144.8416)
  line L651 (208.1216, 144.8416) -> (208.5025, 144.5975)
  spline S5 degree 5 poles (220.5972, 109.701) (220.6772, 109.7589) (220.8371, 109.8747) (221.0769, 110.0484) (221.3966, 110.28) (221.7963, 110.5694) (222.116, 110.801) (222.3559, 110.9747) (222.5157, 111.0905) (222.5957, 111.1484) knots 0 0 0 0 0 0 0.2 0.4 0.6 0.8 1 1 1 1 1 1
  line L652 (208.9, 162.2) -> (211.4718, 161.7435)
  point P0 (233.53, 139.1819)
  point P1 (233.1226, 127.7476)
  point P2 (228.781, 149.6071)
  point P3 (218.3562, 139.7771)
  point P4 (218.3562, 127.7001)
  point P5 (228.8517, 117.4959)
  dimension "d12" = 0.1
  constraint horizontal L582
  constraint vertical L583
  constraint horizontal L584
  constraint vertical L585
  constraint tangent L584 A10
  constraint midpoint S1.end L586
  constraint midpoint L172.start L587
  constraint midpoint L238.start L588
  constraint coincident A7 S3.start
  constraint midpoint S3.start L589
  constraint coincident S2 L238.start
  constraint midpoint L345.end L652
extrude "Extrusion2" add sketch "Esquisse4" along normal blind 2 separate body contours L0 L3 L4 L6 L494 L504 L507 L511 L536 L542 L544 L546 L548 L549 L553 L554 L557 L569 L573 L574 L577 A8 A9 | L20 L22 L26 L28 L35 L37 L38 L40 L41 L44 L46 L49 L50 L51 L59 L63 L91 L113 L257 L289 L291 L292 L293 L294 L295 L298 L299 L300 L302 L303 L306 L307 L308 L309 L313 L315 L316 L319 L321 L326 L328 L329 L331 L333 L334 L360 L420 L451 L458 L472 L473 L474 L479 L487 L489 L490 A2 A3 | L172 L340 L341 L343 L344 L345 L346 L352 L353 L356 L357 L358 L359 L361 L363 L366 L367 L368 L371 L376 L378 L381 L382 L385 L390 L412 A4 S1 L586 S2 L587 S4 | L172 L340 L341 L343 L344 L346 L353 L356 L357 L358 L359 L361 L363 L366 L367 L368 L371 L376 L378 L382 L385 L390 L412 A4 S1 S2 L587 S4 L652 | L586 L587 S4 | L176 L177 L179 L180 L181 L182 L185 L188 L189 L190 L192 L193 L197 A0 L203 L205 L207 L209 L210 L213 L214 L216 L220 L227 L230 L232 L234 L235 L239 L241 L249 L263 L283 L285 A6 A7 S3 | L345 L352 L381 L385 L652 picked at (156.263, 101.7764) makes body 2 at (154.9757, 155.9967, 3) makes body 3 at (203.9727, 88.1107, 1) makes body 4 at (209.0484, 161.8349, 1) makes body 5 at (156.287, 101.7741, 1)
extrude "Extrusion3" add sketch "Esquisse4" along normal blind 4 separate body contours L0 L3 L4 L6 L494 L504 L507 L511 L536 L542 L544 L546 L548 L549 L553 L554 L557 L569 L573 L574 L577 A8 A9 | L1 L2 L5 L7 L8 L9 L10 L11 L12 L13 L14 L15 L16 L17 L18 L19 L23 L29 L31 L34 L36 L43 L45 L47 L48 L50 L55 L58 L60 L61 L62 L409 L415 L417 L419 L422 L426 L427 L435 L438 L439 L441 L442 L443 L447 L448 L449 L450 L452 L453 L454 L455 L456 L457 L460 L461 L463 L464 L466 L467 L468 L469 L470 L471 L475 L476 L477 L478 L480 L481 L482 L483 L484 L485 L488 L490 L491 L496 L497 L499 L502 L507 L509 L513 L514 L515 L516 L517 L519 L520 L521 L523 L524 L525 L526 L528 L531 L532 L538 L539 A3 A8 | L440 L444 L445 L446 L459 L462 L465 L486 L492 L493 L495 L498 L500 L501 L503 L505 L506 L508 L510 L512 L518 L522 L527 L529 L530 L533 L534 L535 L536 L537 L540 L541 L543 L545 L547 L550 L551 L552 L555 L556 L558 L559 L560 L561 L562 L563 L564 L565 L566 L567 L568 L569 L570 L571 L572 L575 L576 L578 L579 L580 L581 A9 | L20 L22 L26 L28 L35 L37 L38 L40 L41 L44 L46 L49 L50 L51 L59 L63 L91 L113 L420 L451 L458 L472 L473 L474 L479 L487 L489 L490 A2 A3 | L21 L24 L25 L27 L30 L32 L33 L38 L39 L42 L52 L54 L56 L57 L64 L65 L66 L68 L69 L71 L72 L74 L76 L78 L79 L80 L81 L82 L83 L84 L85 L86 L88 L89 L90 L91 L92 L93 L94 L95 L96 L97 L98 L99 L100 L101 L102 L103 L105 L106 L107 L109 L111 L112 L114 L115 L120 L129 L130 A2 | L176 L177 L179 L180 L181 L182 L185 L188 L189 L190 L192 L193 L197 A0 L203 L205 L207 L209 L210 L213 L214 L216 L220 L227 L232 L235 L239 L241 L249 L263 L283 L285 A6 A7 S3 | L171 L173 L174 L175 L178 L183 L184 L186 L187 L189 L191 L194 L195 L196 L198 A0 L201 L202 L204 L212 L219 L221 L226 L230 L233 L234 L236 L237 L242 L251 L254 L256 L264 L267 L269 L270 L275 L276 L279 L282 A6 | L53 L67 L70 L73 L75 L77 L87 L108 L116 L117 L118 L119 L122 L123 L124 L125 L126 L127 L128 L131 L133 L134 L135 L136 L138 L139 L142 L143 L144 L145 L146 L147 L148 L149 L150 L153 L154 L155 L157 L158 L159 L161 L163 L165 L166 L167 L168 L170 A5 | L104 L110 L121 L132 L137 L140 L141 L151 L152 L156 L160 L162 L163 L164 L169 L170 A5 picked at (166.6288, 103.1292) picked at (160.0089, 91.9754) picked at (158.3422, 164.8516) picked at (218.2575, 165.6667) makes body 6 at (174.9247, 134.0504, 1) makes body 7 at (210.0652, 101.5384, 5) makes body 8 at (217.8151, 164.8674, 1)
extrude "Extrusion5" add sketch "Esquisse4" along normal blind 4 separate body contours L172 L340 L341 L343 L344 L346 L353 L356 L357 L358 L359 L361 L363 L366 L367 L368 L371 L376 L378 L382 L385 L390 L412 A4 S1 S2 L587 S4 L652 | L345 L352 L381 L385 L652 | L590 L591 L592 L593 L594 L595 L596 L597 L598 L599 L600 L601 L602 L603 A11 L604 L605 L606 L607 L608 L609 L610 L611 L612 L613 L614 L615 L616 L617 L618 L619 L620 L621 L622 L623 L624 L625 L626 L627 L628 L629 L630 L631 L632 L633 L634 L635 L636 L637 L638 L639 L640 L641 L642 L643 L644 L645 L646 L647 L648 L649 L650 L651 makes body 9 at (212.5815, 153.7144, 1) makes body 10 at (202.4776, 140.6317, 1)
extrude "Extrusion7" add sketch "Esquisse4" along normal blind 4 separate body contours L199 L200 L206 L208 L210 L211 L215 L217 L218 L222 L223 L224 L225 L228 L229 L231 L240 L243 L244 L245 L246 L247 L248 L250 L252 L253 L255 L258 L259 L260 L261 L262 L265 L266 L268 L271 L272 L273 L274 L277 L278 L280 L281 L284 L286 L287 L288 L290 L296 L297 L301 L303 L304 L305 L310 L311 L312 L314 L317 L318 L319 L320 L322 L323 L324 L325 L327 L330 L332 L335 L336 L359 L380 L383 A3 A4 A7 S0 S2 S5 makes body 11
combine "Combiner1" operation add target body 11 tool bodies 9
extrude "Extrusion8" add sketch "Esquisse4" along normal blind 4 contours L257 L289 L291 L292 L293 L294 L295 L298 L299 L300 L302 L303 L306 L307 L308 L309 L313 L315 L316 L319 L321 L326 L328 L329 L331 L333 L334 L360 A3 bodies 11
sketch "Esquisse5" plane through (0, 0, 0) normal (0, 0, 1) x (1, 0, 0)
sketch "Esquisse6" plane through (0, 0, 1) normal (0, 0, 1) x (1, 0, 0)
  circle A0 centre (187.25, 129.75) radius 89.75
extrude "Extrusion9" add sketch "Esquisse6" along normal blind 0.2 separate body makes body 12
combine "Combiner2" operation add target body 7 tool bodies 11
delete_body "RemoveBody1" bodies 1
extrude "Extrusion6" add sketch "Esquisse4" along normal blind 4 separate body contours L199 L200 L206 L208 L210 L211 L215 L217 L218 L222 L223 L224 L225 L228 L229 L231 L240 L243 L244 L245 L246 L247 L248 L250 L252 L253 L255 L258 L259 L260 L261 L262 L265 L266 L268 L271 L272 L273 L274 L277 L278 L280 L281 L284 L286 L287 L288 L290 L296 L297 L301 L303 L304 L305 L310 L311 L312 L314 L317 L318 L319 L320 L322 L323 L324 L325 L327 L330 L332 L335 L336 L359 L380 L383 A3 A4 A7 S0 S2 S5 makes body 13
extrude "Extrusion4" add sketch "Esquisse4" along normal blind 4 separate body contours L590 L591 L592 L593 L594 L595 L596 L597 L598 L599 L600 L601 L602 L603 A11 L604 L605 L606 L607 L608 L609 L610 L611 L612 L613 L614 L615 L616 L617 L618 L619 L620 L621 L622 L623 L624 L625 L626 L627 L628 L629 L630 L631 L632 L633 L634 L635 L636 L637 L638 L639 L640 L641 L642 L643 L644 L645 L646 L647 L648 L649 L650 L651 makes body 14
extrude "Extrusion10" cut 4 faces at (209.0484, 161.8349, 3) (154.9757, 155.9967, 3) (203.9727, 88.1107, 3) (156.287, 101.7741, 3) along direction (0, 0, -1) blind 20 on bodies 2 3 4 5 bodies 7 12 makes body 15 at (219.1747, 167.6513, 1)
extrude "Extrusion11" add sketch "Esquisse6" along normal blind 0.2 separate body makes body 16
combine "Combiner3" operation add target body 7 tool bodies 13
hidden bodies 16
named bodies: "TopLeftCircle", "DownRightCircle", "TopRightCircle", "DownLeftCircle", "LeftDroneArmature", "XTopRight", "XMidRIght", "TopLeftInnerCircle (1)", "TopLeftInnerCircle", "CircleBg"
